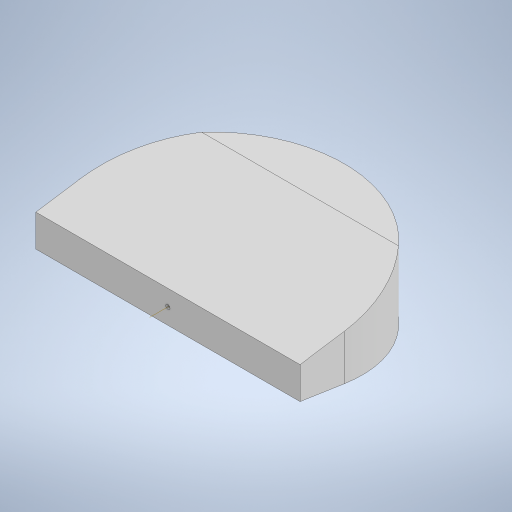
# Autodesk Inventor part: Сыр
Saved by Autodesk Inventor 2023.2 (Build 272271030, 271C)
## iProperties
Created: 2024-01-31
Part Number: Сыр
Material: Типовые
Document SubType Name: Modeling
Designer: I9232
Density: 1 g/cm^3
Appearance: По умолчанию
Author: I9232
Autodesk Inventor part; units mm, degrees
ref_plane "YZ Plane" through (0, 0, 0) normal (1, 0, 0) x (0, 1, 0)
ref_plane "XZ Plane" through (0, 0, 0) normal (0, 1, 0) x (-1, 0, 0)
ref_plane "XY Plane" through (0, 0, 0) normal (0, 0, 1) x (1, 0, 0)
sketch "Эскиз1" plane through (0, 0, 0) normal (0, 1, 0) x (-1, 0, 0)
  line L0 (165, 0.2529) -> (-165, 0.2529)
  line L1 (-165, 0.2529) -> (-165, -54.7471)
  line L2 (165, 0.2529) -> (165, -54.7471)
  arc A0 (-165, -54.7471) -> (165, -54.7471) centre (0, -54.7471) ccw
  point P0 (0, 0)
  dimension "d1" = 330
  dimension "d5" = 55
  dimension "d8" = 55
  constraints: 6 end point, 2 point on circle, 2 tangent, 2 vertical, 1 centre point
  measures "d1" distance of L0.start L0.end
  measures "d5" distance of L0.end L1.end
  measures "d8" distance of L0.start L2.end
extrude "Выдавливание1" add sketch "Эскиз1" along normal mid plane 90
sketch "Эскиз2" plane through (0, 0, 0) normal (1, 0, 0) x (0, 1, 0)
  line L0 (-45, -54.7471) -> (45, -54.7471) projected
  line L1 (45, 0.2529) -> (45, -54.7471) projected
  line L2 (0, -101.1017) -> (0, -121.0064)
  line L3 (-20, -219.7471) -> (-45, -54.7471)
  line L4 (20, 0.2529) -> (45, -164.7471)
  line L5 (45, 0.2529) -> (20, 0.2529)
  line L6 (45, 0.2529) -> (45, -164.7471)
  line L7 (-45, 0.2529) -> (-45, -54.7471)
  line L8 (-20, 0.2529) -> (-45, -164.7471)
  line L9 (-45, 0.2529) -> (-20, 0.2529)
  line L10 (-45, 0.2529) -> (-45, -164.7471)
  point P0 (0, 0)
  constraints: 18 end point, 3 symmetric about line, 1 horizontal, 1 perpendicular, 1 vertical
extrude "Выдавливание2" cut sketch "Эскиз2" along normal mid plane 330
sketch "Эскиз3" plane through (-165, -20, 0.2529) normal (0, 0, 1) x (1, 0, 0)
  circle A0 centre (165, 20) radius 2.65
  dimension "d14" = 5.3
  constraints: 1 centre point, 1 coincident
  measures "d14" diameter of A0
extrude "Выдавливание3" cut sketch "Эскиз3" against normal up to surface
